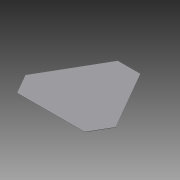
# Autodesk Inventor part: Top Plate
Saved by Autodesk Inventor 2013 (Build 170138000, 138)
## iProperties
Created: 2013-01-12
Part Number: Top Plate
Material: Generic
Document SubType Name: Modeling
Designer: carneeki
Density: 1 g/cm^3
Author: carneeki
Autodesk Inventor part; units mm, degrees
ref_plane "YZ Plane" through (0, 0, 0) normal (1, 0, 0) x (0, 1, 0)
ref_plane "XZ Plane" through (0, 0, 0) normal (0, 1, 0) x (-1, 0, 0)
ref_plane "XY Plane" through (0, 0, 0) normal (0, 0, 1) x (1, 0, 0)
sketch "Sketch1" plane through (0, 0, 0) normal (0, 1, 0) x (-1, 0, 0)
  line L0 (304.8, 351.9527) -> (-304.8, 351.9527)
  line L1 (-304.8, 351.9527) -> (-406.4, 175.9764)
  line L2 (-406.4, 175.9764) -> (-101.6, -351.9527)
  line L3 (-101.6, -351.9527) -> (101.6, -351.9527)
  line L4 (101.6, -351.9527) -> (406.4, 175.9764)
  line L5 (406.4, 175.9764) -> (304.8, 351.9527)
  line L6 (-254, -87.9882) -> (0, 58.6588) construction
  line L7 (254, -87.9882) -> (0, 58.6588) construction
  line L8 (0, 351.9527) -> (0, 58.6588) construction
  point P0 (-355.6, 263.9645)
  dimension "d0" = 609.6
  dimension "d1" = 203.2
  dimension "d2" = 120
  dimension "d3" = 609.6
  dimension "d4" = 120
  dimension "d5" = 203.2
  dimension "d6" = 240
  dimension "d7" = 609.6
  dimension "d8" = 120
  dimension "d9" = 203.2
  dimension "d10" = 120
  dimension "d16" = 293.2939
  dimension "d17" = 120
  dimension "d18" = 120
  dimension "d19" = 120
  constraints: 18 end point, 4 midpoint, 2 parallel, 1 horizontal, 1 perpendicular
  measures "d0" distance of L0.start L0.end
  measures "d1" distance of L0.end L1.end
  measures "d2" angle of L1 L0
  measures "d3" distance of L1.end L2.end
  measures "d4" angle of L2 L1
  measures "d5" distance of L2.end L3.end
  measures "d7" distance of L3.end L4.end
  measures "d8" angle of L4 L3
  measures "d9" distance of L4.end L0.start
  measures "d10" angle of L5 L4
  measures "d16" distance of L8.start L6.end
  measures "d17" angle of L8 L6
  measures "d18" angle of L6 L7
  measures "d19" angle of L8 L7
extrude "Extrusion1" add sketch "Sketch1" against normal blind 3
body "Solid1"
